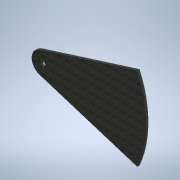
# Autodesk Inventor part: pendulumCompound
Saved by Autodesk Inventor 2020 (Build 240168000, 168)
## iProperties
Created: 2020-06-14
Part Number: pendulumCompound
Material: Steel
Document SubType Name: Modeling
Designer: Freeman
Mass: 1.07551e+06 g
Surface Area: 58450.5 cm^2
Volume: 137008 cm^3
Density: 7.85 g/cm^3
Appearance: Plate
Author: Freeman
Autodesk Inventor part; units mm, degrees
ref_plane "YZ Plane" through (0, 0, 0) normal (1, 0, 0) x (0, 1, 0)
ref_plane "XZ Plane" through (0, 0, 0) normal (0, 1, 0) x (-1, 0, 0)
ref_plane "XY Plane" through (0, 0, 0) normal (0, 0, 1) x (1, 0, 0)
sketch "Sketch3" plane through (0, 0, 0) normal (0, 0, 1) x (1, 0, 0)
  circle A0 centre (0, 0) radius 50
  arc A1 (-75.1764, 238.4292) -> (-75.1764, -238.4292) centre (0, 0) ccw
  arc A2 (2057.3995, -910.8278) -> (2057.3995, 910.8278) centre (0, 0) ccw
  line L0 (-75.1764, 238.4292) -> (2057.3995, 910.8278)
  line L1 (-75.1764, -238.4292) -> (2057.3995, -910.8278)
  line L2 (0, 0) -> (2250, 0)
  dimension "d8" = 100
  dimension "d9" = 500
  dimension "d10" = 4500
  dimension "d11" = 35
  constraints: 6 end point, 5 point on circle, 3 centre point, 3 coincident, 2 tangent, 1 horizontal
  measures "d8" diameter of A0
  measures "d9" diameter of A1
  measures "d10" diameter of A2
  measures "d11" angle of L1 L0
extrude "Extrusion1" add sketch "Sketch3" along normal mid plane 50
body "Solid1"
